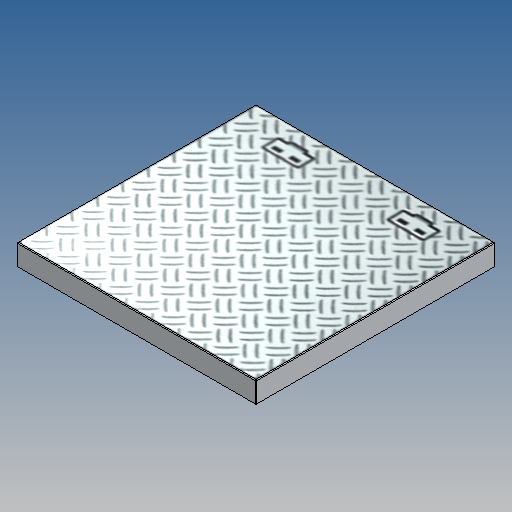
# Autodesk Inventor part: 42146_1751_1
Saved by Autodesk Inventor 2025 (Build 290162010, 162A)
## iProperties
Created: 2014-06-03
Part Number: 42146_1751_1
Material: ABS Plastic
Document SubType Name: Modeling
Designer: D. Kohfeld
Density: 1.06 g/cm^3
Appearance: LtBluishGray
Mass: 0.889134 g
Surface Area: 12.4005 cm^2
Volume: 0.838805 cm^3
Author: D. Kohfeld
Autodesk Inventor part; units mm, degrees
ref_plane "YZ Plane" through (0, 0, 0) normal (1, 0, 0) x (0, 1, 0)
ref_plane "XZ Plane" through (0, 0, 0) normal (0, 1, 0) x (-1, 0, 0)
ref_plane "XY Plane" through (0, 0, 0) normal (0, 0, 1) x (1, 0, 0)
sketch "Sketch2" plane through (0, 0, 0) normal (0, 1, 0) x (-1, 0, 0)
  line L0 (-16, 16) -> (16, 16)
  line L1 (16, 16) -> (16, -16)
  line L2 (16, -16) -> (-16, -16)
  line L3 (-16, -16) -> (-16, 16)
  point P0 (0, 0)
  point P1 (0, 16)
  point P2 (-16, 0)
  dimension "d0" = 32
  dimension "d1" = 32
  constraints: 8 end point, 2 midpoint, 2 parallel, 1 horizontal, 1 horizontal alignment, 1 perpendicular, 1 vertical alignment
  measures "d0" distance of L1.end L2.end
  measures "d1" distance of L2.end L0.start
extrude "Extrusion1" add sketch "Sketch2" along normal blind 3.2
sketch "Sketch3" plane through (0, 0, 0) normal (0, -1, 0) x (1, 0, 0)
  line L0 (-16, 16) -> (-16, -16) projected
  line L1 (-14.4, 14.4) -> (14.4, 14.4)
  line L2 (14.4, 14.4) -> (14.4, -14.4)
  line L3 (14.4, -14.4) -> (-14.4, -14.4)
  line L4 (-14.4, -14.4) -> (-14.4, 14.4)
  circle A0 centre (-8, 0) radius 3.2569
  circle A1 centre (-8, 0) radius 2.4
  line L5 (-16, -16) -> (16, -16) projected
  circle A2 centre (0, 0) radius 1.6
  line L6 (16, -16) -> (16, 16) projected
  line L7 (-12, 0) -> (-4, 0) construction
  line L8 (-4, 0) -> (4, 0) construction
  line L9 (4, 0) -> (12, 0) construction
  circle A3 centre (-12, 12) radius 2.4 construction
  circle A4 centre (-12, -12) radius 2.4 construction
  circle A5 centre (12, -12) radius 2.4 construction
  circle A6 centre (12, 12) radius 2.4 construction
  line L10 (16, 16) -> (-16, 16) projected
  line L11 (-15.6, 15.6) -> (15.6, 15.6)
  line L12 (15.6, 15.6) -> (15.6, -15.6)
  line L13 (15.6, -15.6) -> (-15.6, -15.6)
  line L14 (-15.6, -15.6) -> (-15.6, 15.6)
  circle A7 centre (-12, 4) radius 2.4 construction
  point P0 (-14.4, 0)
  point P1 (0, 14.4)
  point P2 (0, 0)
  point P3 (0, 15.6)
  point P4 (-15.6, 0)
  dimension "d61" = 4.8
  dimension "d75" = 8
  dimension "d76" = 16
  dimension "d86" = 3.2
  dimension "d92" = 8
  dimension "d98" = 24
  dimension "d99" = 24
  dimension "d102" = 0.4
  dimension "d103" = 0.4
  dimension "d106" = 8
  constraints: 22 end point, 10 tangent, 8 centre point, 6 equal length, 5 midpoint, 4 equal radius, 3 coincident, 3 perpendicular, 3 vertical alignment, 2 collinear, 2 horizontal, 2 horizontal alignment
  measures "d61" diameter of A1
  measures "d75" distance from line of A0.centre L0
  measures "d76" distance from line of A0.centre L5
  measures "d86" diameter of A2
  measures "d92" distance of L7.end L8.end
  measures "d98" distance of A6.centre A3.centre
  measures "d99" distance of A4.centre A3.centre
  measures "d102" distance between parallel lines of L11 L10
  measures "d103" distance between parallel lines of L0 L14
  measures "d106" distance of A3.centre A7.centre
extrude "Extrusion2" cut sketch "Sketch3" against normal blind 1.6 contours L1 L2 L3 L4 | A0 | A1 | A2
extrude "Extrusion7" cut sketch "Sketch3" against normal blind 0.4 contours L10 L6 L5 L0
extrude "Extrusion6" add sketch "Sketch3" against normal up to next contours A0
pattern_linear "Rectangular Pattern3" count 3 spacing 8 along (1, 0, 0) count 3 spacing 8 along (0, 0, -1) of "Extrusion6" second direction both ways yes
fillet "Fillet1" radius 0.1 8 edges at (-16, 1.8, 16) (0, 3.2, 16) (-16, 3.2, 0) (16, 1.8, 16) (16, 3.2, 0) (0, 3.2, -16) (16, 1.8, -16) (-16, 1.8, -16)
sketch "Skizze10" plane through (0, 3.2, 0) normal (0, 1, 0) x (1, 0, 0)
  line L0 (-15.9, 15.9) -> (15.9, 15.9) projected
  line L1 (-16.3705, 16.4) -> (16.3705, 16.4) construction
  line L2 (16.3705, 16.4) -> (16.3705, -16.4) construction
  line L3 (16.3705, -16.4) -> (-16.3705, -16.4) construction
  line L4 (-16.3705, -16.4) -> (-16.3705, 16.4) construction
  point P0 (0, 0)
  point P1 (0, 16.4)
  point P2 (-16.3705, 0)
  dimension "d123" = 0.5
  constraints: 2 midpoint, 1 horizontal, 1 horizontal alignment, 1 vertical alignment, 2 other
  measures "d123" distance between parallel lines of L0 L1
decal "Aufkleber1"
equation "\"d4\" = 0.333333 * lh"
equation "\"d61\" = kd"
equation "\"d75\" = lu"
equation "\"d76\" = 2 * d75"
equation "\"d86\" = pd"
equation "\"d92\" = lu"
equation "\"d98\" = d99"
equation "\"d99\" = 3 * d75"
equation "\"d102\" = gw"
equation "\"d103\" = gw"
equation "\"d106\" = lu"
equation "\"d11\" = 0.333333 * lh - topthk"
equation "\"d104\" = gh"
equation "\"d91\" = lu"
equation "\"d109\" = lu"
equation "\"d22\" = lf"
equation "\"lh\" = 9.6"
equation "\"kd\" = 4.8"
equation "\"lu\" = 8"
equation "\"pd\" = 3.2"
equation "\"gw\" = 0.4"
equation "\"topthk\" = 1.6"
equation "\"gh\" = 0.4"
equation "\"lf\" = 0.1"
body "Solid1"
